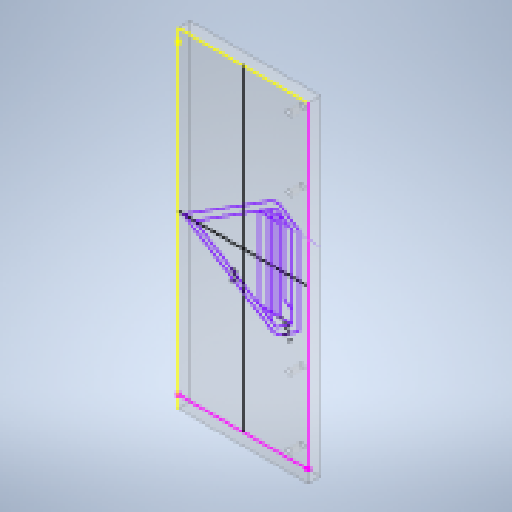
# Autodesk Inventor part: 부품76
Saved by Autodesk Inventor 2024 (Build 280153000, 153)
## iProperties
Created: 2024-09-09
Part Number: 부품76
Material: PMMA 플라스틱
Document SubType Name: Modeling
Designer: Eungang
Mass: 122.709 g
Surface Area: 253.571 cm^2
Volume: 103.29 cm^3
Density: 1.188 g/cm^3
Appearance: 폴리카보네이트 - 선명
Author: Eungang
Autodesk Inventor part; units mm, degrees
ref_plane "YZ Plane" through (0, 0, 0) normal (1, 0, 0) x (0, 1, 0)
ref_plane "XZ Plane" through (0, 0, 0) normal (0, 1, 0) x (-1, 0, 0)
ref_plane "XY Plane" through (0, 0, 0) normal (0, 0, 1) x (1, 0, 0)
sketch "스케치1" plane through (0, 0, 0) normal (0, 0, 1) x (1, 0, 0)
  line L0 (0, 0) -> (63.841, 0) projected
  line L1 (63.841, 0) -> (63.841, 6) projected
  line L2 (0, 6) -> (63.841, 6) projected
  line L3 (0, 0) -> (0, 6) projected
  circle A0 centre (54.8408, -3) radius 1.45 projected
  line L4 (63.841, 0) -> (51.8408, 0) projected
  line L5 (51.8408, 0) -> (51.8408, -12) projected
  line L6 (51.8408, -12) -> (57.8409, -12) projected
  line L7 (57.8409, -12) -> (57.8409, -6) projected
  line L8 (57.8409, -6) -> (63.841, -6) projected
  line L9 (63.841, -6) -> (63.841, 0) projected
  line L10 (46.0408, 0) -> (46.0408, -150) projected
  line L11 (63.841, 6) -> (0, 6)
  line L12 (0, 6) -> (0, -150)
  line L13 (0, -150) -> (63.841, -150)
  line L14 (63.841, -150) -> (63.841, 6)
  line L15 (63.841, -75) -> (51.8408, -75)
  circle A1 centre (54.8408, -147) radius 1.45
  line L16 (63.841, -150) -> (51.8408, -150)
  line L17 (51.8408, -150) -> (51.8408, -138)
  line L18 (51.8408, -138) -> (57.8409, -138)
  line L19 (57.8409, -138) -> (57.8409, -144)
  line L20 (57.8409, -144) -> (63.841, -144)
  line L21 (63.841, -144) -> (63.841, -150)
  line L22 (1.1205, -156.4) -> (64.9491, -156.4) projected
  line L23 (64.9491, -156.4) -> (64.9491, -150.4) projected
  line L24 (1.1205, -150.4) -> (64.9491, -150.4) projected
  line L25 (1.1205, -156.4) -> (1.1205, -150.4) projected
  line L26 (63.841, -150) -> (63.841, -156)
  line L27 (0, -150) -> (0, -156)
  line L28 (63.841, -156) -> (0, -156)
  line L29 (63.841, -156) -> (0, -156)
  line L30 (0, -156) -> (0, -156.4)
  line L31 (0, -156.4) -> (63.841, -156.4)
  line L32 (63.841, -156.4) -> (63.841, -156)
  line L33 (5.8, -150) -> (5.8, 0) projected
  line L34 (46.0408, -150) -> (51.8408, -150) projected
  line L35 (51.8408, -150) -> (51.8408, 0) projected
  line L36 (51.8408, 0) -> (46.0408, 0) projected
  line L37 (0, 0) -> (0, -150) projected
  line L38 (0, -150) -> (5.8, -150) projected
  line L39 (5.8, 0) -> (0, 0) projected
  point P0 (0, -156)
  point P1 (1.1205, -156)
  point P2 (0, -156)
  constraints: 36 end point, 8 symmetric about line, 4 parallel, 2 horizontal, 2 perpendicular, 1 centre point, 1 point on line, 1 other
extrude "돌출1" add sketch "스케치1" along normal blind 6 contours L3 L2 L1 L0 | L0 L33 L13 L12 | L0 L10 L13 L33 | L13 L26 L24 L25 L28 L27 | L0 L5 L35 L17 L13 L10 | L0 L9 L8 L7 L6 L5 | L25 L24 L26 L28 | L6 L7 L8 L14 L15 L35 | L17 L18 L19 L20 L14 L13 | L15 L14 L20 L19 L18 L35 | A0 | A1
sketch "스케치2" plane through (0, 0, 6) normal (0, 0, 1) x (1, 0, 0)
  line L0 (63.841, 6) -> (0, 6) projected
  line L1 (31.9205, 6) -> (31.9205, -150)
  line L2 (0, -150) -> (63.841, -150) projected
  line L3 (63.841, -150) -> (63.841, 6) projected
  line L4 (63.841, -72) -> (0, -72)
  line L5 (0, 6) -> (0, -156) projected
  line L6 (31.9205, -72) -> (0, -72)
  line L7 (63.841, -72) -> (31.9205, -72)
  line L8 (47.8807, -72) -> (15.9603, -72)
  line L9 (47.8807, -52) -> (70.452, -52) construction
  line L10 (0, -72) -> (15.9603, -72)
  line L11 (55.9312, -52.0469) -> (55.8609, -92)
  line L12 (31.9205, -72) -> (47.8807, -72)
  line L13 (47.909, -97.3012) -> (7.9801, -72)
  line L14 (47.909, -46.6988) -> (7.9801, -72)
  line L15 (47.909, -97.3012) -> (55.8609, -92)
  line L16 (55.9312, -52.0469) -> (47.909, -46.6988)
  line L17 (49.5449, -99.8162) -> (58.858, -93.6074)
  line L18 (58.858, -93.6074) -> (58.9341, -50.4432)
  line L19 (58.9341, -50.4432) -> (49.5449, -44.1838)
  line L20 (46.2731, -99.8162) -> (2.3752, -72)
  line L21 (2.3752, -72) -> (46.2731, -44.1838)
  line L22 (46.2731, -44.1838) -> (49.5449, -44.1838)
  line L23 (49.5449, -99.8162) -> (46.2731, -99.8162)
  line L24 (55.8715, -85.95) -> (51.8815, -83.2899)
  line L25 (51.8815, -83.2899) -> (51.9201, -49.3728)
  line L26 (55.8609, -92) -> (47.8807, -92)
  line L27 (51.9201, -49.3728) -> (43.6889, -49.3728)
  line L28 (43.6889, -49.3728) -> (43.6889, -94.6272)
  line L29 (39.5429, -52) -> (43.6889, -52)
  line L30 (43.6889, -52) -> (43.6889, -92)
  line L31 (43.6889, -92) -> (39.5429, -92)
  line L32 (39.5429, -92) -> (39.5429, -52)
  line L33 (49.5449, -49.3728) -> (49.5449, -92)
  line L34 (47.8045, -49.3728) -> (43.6889, -49.3728)
  line L35 (45.7467, -49.3728) -> (45.7467, -95.9311)
  line L36 (43.6889, -52) -> (49.5449, -52)
  line L37 (39.5429, -92) -> (43.6889, -92)
  line L38 (43.6889, -92) -> (43.6889, -52)
  line L39 (43.6889, -52) -> (39.5429, -52)
  line L40 (39.5429, -52) -> (39.5429, -92)
  line L41 (47.8807, -92) -> (43.6889, -92)
  line L42 (47.8807, -92) -> (47.8807, -49.3728)
  point P0 (0, 0)
  dimension "d4" = 3
  dimension "d5" = 3
  constraints: 78 end point, 13 point on line, 10 midpoint, 9 perpendicular, 7 parallel, 5 horizontal, 2 collinear, 3 other
  measures "d4" distance between parallel lines of L15 L17
  measures "d5" distance between parallel lines of L13 L20
sketch "스케치3" plane through (0, 0, 6) normal (0, 0, 1) x (1, 0, 0)
  point P0 (0, 0)
sketch "스케치4" plane through (0, 0, 6) normal (0, 0, 1) x (1, 0, 0)
  circle A0 centre (54.8408, -36.9997) radius 1.35 projected
  line L0 (51.8408, -33.9997) -> (51.8408, -39.9997) projected
  line L1 (51.8408, -39.9997) -> (102.8408, -39.9997) projected
  line L2 (102.8408, -33.9997) -> (102.8408, -39.9997) projected
  line L3 (51.8408, -33.9997) -> (102.8408, -33.9997) projected
  circle A1 centre (54.8408, -113.3997) radius 1.35 projected
  line L4 (51.8408, -110.3997) -> (51.8408, -116.3997) projected
  line L5 (51.8408, -116.3997) -> (102.8408, -116.3997) projected
  line L6 (102.8408, -116.3997) -> (102.8408, -110.3997) projected
  line L7 (51.8408, -110.3997) -> (102.8408, -110.3997) projected
  point P0 (0, 0)
extrude "돌출2" cut sketch "스케치4" against normal blind 10 contours A0 | A1
sketch "스케치6" plane through (0, 0, 0) normal (0, 0, -1) x (-1, 0, 0)
  circle A0 centre (-55.0408, -146.8) radius 1.35 projected
  line L0 (-52.0408, -149.8) -> (-52.0408, -137.8) projected
  line L1 (-52.0408, -149.8) -> (-64.0408, -149.8) projected
  line L2 (-64.0408, -149.8) -> (-64.0408, -143.8) projected
  line L3 (-58.0408, -143.8) -> (-64.0408, -143.8) projected
  line L4 (-58.0408, -143.8) -> (-58.0408, -137.8) projected
  line L5 (-52.0408, -137.8) -> (-58.0408, -137.8) projected
  circle A1 centre (-55.5547, -3.2) radius 1.35 projected
  line L6 (-52.5547, -0.2) -> (-52.5547, -12.2) projected
  line L7 (-52.5547, -12.2) -> (-58.5547, -12.2) projected
  line L8 (-58.5547, -6.2) -> (-58.5547, -12.2) projected
  line L9 (-58.5547, -6.2) -> (-64.5547, -6.2) projected
  line L10 (-64.5547, -0.2) -> (-64.5547, -6.2) projected
  line L11 (-52.5547, -0.2) -> (-64.5547, -0.2) projected
  point P0 (0, 0)
extrude "돌출4" cut sketch "스케치6" against normal up to next contours A0 | A1
